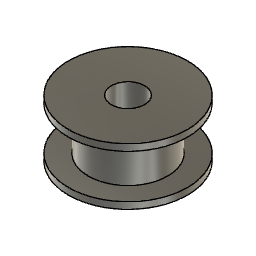
PoleaLUKEN v1 (Autodesk Fusion 360 design; units mm, degrees)
Autodesk Fusion 360 part; units mm, degrees
cylinder "CilindroPrimitivo1" add diameter 18 height 1 placed x (1, 0, 0) y (0, 1, 0) z (0, 0, 1) at (0, 0, 0)
cylinder "CilindroPrimitivo2" add diameter 12 height 8.6 placed x (1, 0, 0) y (0, 1, 0) z (0, 0, 1) at (0, 0, 1)
delete_face "SuprimirCaras1" 1 faces at (5.9702, -0.5974, 3.8667)
cylinder "CilindroPrimitivo3" add diameter 12 height 6.6 placed x (1, 0, 0) y (0, 1, 0) z (0, 0, 1) at (0, 0, 1)
cylinder "CilindroPrimitivo4" add diameter 18 height 1 placed x (1, 0, 0) y (0, 1, 0) z (0, 0, 1) at (0, 0, 7.6)
sketch "Boceto7" plane through (0, 0, 8.6) normal (0, 0, 1) x (-1, 0, 0)
  circle A0 centre (0, 0) radius 9
  circle A1 centre (0, 0) radius 2.5
  dimension "d27" = 5
  constraint coincident A0.centre A1.centre
  measures "d27" diameter of A1
extrude "Extruir3" cut sketch "Boceto7" against normal blind 13 contours A1
move_body "Desplazar1" bodies 1 to x (1, 0, 0) y (0, 1, 0) z (0, 0, 1) at (0, 0, 2)
move_body "Desplazar2" bodies 1 to x (1, 0, 0) y (0, 1, 0) z (0, 0, 1) at (-2, 0, 0)
move_body "Desplazar3" bodies 1 to x (1, 0, 0) y (0, 1, 0) z (0, 0, 1) at (4, 0, -2)
move_body "Desplazar4" bodies 1 to x (1, 0, 0) y (0, 1, 0) z (0, 0, 1) at (-2, 0, 0)
equation "LonX = 40 mm"
equation "LonY = 30 mm"
equation "LonZ = 50 mm"
equation "Prof202 = 20 mm"
equation "esp = 5 mm"
equation "DiaPol = 18 mm"
equation "AltPol = 8.6 mm"
equation "tol0 = 1 mm"
equation "M5 = 5 mm"
equation "DiaD = 12 mm"
equation "espPol = 1 mm"
equation "d18 = espPol"
equation "d20 = AltPol"
equation "AltIn = AltPol - ( 2 * espPol )"
equation "d23 = AltIn"
equation "d25 = espPol"
equation "d27 = M5"
